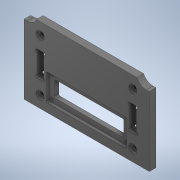
# Autodesk Inventor part: Cockpit_horizontal_frame_05
Saved by Autodesk Inventor 2020.4 (Build 244396000, 396)
## iProperties
Created: 2021-08-14
Part Number: Cockpit_horizontal_frame_05
Material: アセタール樹脂、黒
Document SubType Name: Modeling
Designer: Masato Kubotera
Density: 1.425 g/cm^3
Appearance: 滑らか - 黒
Mass: 37.8231 g
Surface Area: 126.929 cm^2
Volume: 26.5425 cm^3
Description: POM T5
Author: Masato Kubotera
Title: Cockpit_horizontal_frame_05
Autodesk Inventor part; units mm, degrees
ref_plane "YZ Plane" through (0, 0, 0) normal (1, 0, 0) x (0, 1, 0)
ref_plane "XZ Plane" through (0, 0, 0) normal (0, 1, 0) x (-1, 0, 0)
ref_plane "XY Plane" through (0, 0, 0) normal (0, 0, 1) x (1, 0, 0)
sketch "スケッチ1" plane through (0, 0, 0) normal (0, 0, 1) x (1, 0, 0)
  line L0 (-47, 28.25) -> (-37.7144, 28.25)
  line L1 (47, 28.25) -> (47, 23.75)
  line L2 (47, -28.25) -> (-47, -28.25)
  line L3 (-47, -28.25) -> (-47, -11.5167)
  line L4 (-47, 28.25) -> (47, -28.25) construction
  line L5 (47, 28.25) -> (-47, -28.25) construction
  line L6 (0, 28.25) -> (0, -28.25) construction
  line L7 (-47, 11.5167) -> (-47, 23.75)
  line L8 (-47, -11.5167) -> (-47, 11.5167)
  line L9 (47, 11.5167) -> (47, -11.5167)
  line L10 (47, -11.5167) -> (47, -28.25)
  line L11 (-47, 0) -> (47, 0) construction
  arc A0 (-47, 24.0838) -> (-37.7144, 28.25) centre (-44.75, 31.5) ccw
  arc A1 (37.7144, 28.25) -> (47, 24.0838) centre (44.75, 31.5) ccw
  line L12 (-47, 24.0838) -> (-47, 28.25)
  line L13 (-37.7144, 28.25) -> (47, 28.25)
  arc A2 (-37.7144, 28.25) -> (-47, 24.0838) centre (-44.75, 31.5) ccw
  arc A3 (47, 24.0838) -> (37.7144, 28.25) centre (44.75, 31.5) ccw
  line L14 (-44.75, 23.75) -> (-47, 23.75)
  line L15 (44.75, 23.75) -> (47, 23.75)
  line L16 (-47, 23.75) -> (-47, 24.0838)
  line L17 (47, 23.75) -> (47, 11.5167)
  line L18 (-30, -1.75) -> (30, -1.75) construction
  line L19 (30, -1.75) -> (30, -21.75) construction
  line L20 (30, -21.75) -> (-30, -21.75) construction
  line L21 (-30, -21.75) -> (-30, -1.75) construction
  line L22 (-30, -1.75) -> (30, -21.75) construction
  line L23 (30, -1.75) -> (-30, -21.75) construction
  circle A4 centre (-28, -3.75) radius 1.05
  line L24 (30, -11.75) -> (-30, -11.75) construction
  circle A5 centre (-28, -19.75) radius 1.05
  circle A6 centre (28, -3.75) radius 1.05
  circle A7 centre (28, -19.75) radius 1.05
  line L25 (-30.05, -1.7) -> (30.05, -1.7)
  line L26 (30.05, -1.7) -> (30.05, -21.8)
  line L27 (30.05, -21.8) -> (-30.05, -21.8)
  line L28 (-30.05, -21.8) -> (-30.05, -1.7)
  line L29 (-30.05, -1.7) -> (30.05, -21.8) construction
  line L30 (30.05, -1.7) -> (-30.05, -21.8) construction
  line L31 (-26, -5.75) -> (26, -5.75)
  line L32 (26, -5.75) -> (26, -17.75)
  line L33 (26, -17.75) -> (-26, -17.75)
  line L34 (-26, -17.75) -> (-26, -5.75)
  line L35 (-26, -5.75) -> (26, -17.75) construction
  line L36 (26, -5.75) -> (-26, -17.75) construction
  line L37 (-37.25, 9.4167) -> (-32.25, 9.4167) construction
  line L38 (-32.25, 9.4167) -> (-32.25, -9.4167) construction
  line L39 (-32.25, -9.4167) -> (-37.25, -9.4167) construction
  line L40 (-37.25, -9.4167) -> (-37.25, 9.4167) construction
  line L41 (-37.25, 9.4167) -> (-32.25, -9.4167) construction
  line L42 (-32.25, 9.4167) -> (-37.25, -9.4167) construction
  line L43 (-37.26, 9.4267) -> (-32.24, 9.4267)
  line L44 (-32.24, 9.4267) -> (-32.24, 7.3267) construction
  line L45 (-32.24, -9.4267) -> (-37.26, -9.4267)
  line L46 (-37.26, -9.4267) -> (-37.26, -7.3267) construction
  line L47 (-37.26, 9.4267) -> (-32.24, -9.4267) construction
  line L48 (-32.24, 9.4267) -> (-37.26, -9.4267) construction
  arc A8 (-37.26, 9.4267) -> (-37.26, 7.3267) centre (-37.26, 8.3767) ccw
  line L49 (-34.75, 9.4167) -> (-34.75, -9.4167) construction
  line L50 (-37.25, 0) -> (-32.25, 0) construction
  arc A9 (-32.24, 7.3267) -> (-32.24, 9.4267) centre (-32.24, 8.3767) ccw
  arc A10 (-37.26, -7.3267) -> (-37.26, -9.4267) centre (-37.26, -8.3767) ccw
  arc A11 (-32.24, -9.4267) -> (-32.24, -7.3267) centre (-32.24, -8.3767) ccw
  line L51 (-37.26, 7.3267) -> (-37.26, 9.4267) construction
  line L52 (-32.24, 7.3267) -> (-32.24, -7.3267)
  line L53 (-37.26, -7.3267) -> (-37.26, 7.3267)
  line L54 (-32.24, -7.3267) -> (-32.24, -9.4267) construction
  line L55 (37.25, 9.4167) -> (32.25, 9.4167) construction
  line L56 (32.25, 9.4167) -> (32.25, -9.4167) construction
  line L57 (32.25, -9.4167) -> (37.25, -9.4167) construction
  line L58 (37.25, -9.4167) -> (37.25, 9.4167) construction
  line L59 (37.25, 9.4167) -> (32.25, -9.4167) construction
  line L60 (32.25, 9.4167) -> (37.25, -9.4167) construction
  line L61 (37.26, 9.4267) -> (32.24, 9.4267)
  line L62 (32.24, 9.4267) -> (32.24, 7.3267) construction
  line L63 (32.24, -9.4267) -> (37.26, -9.4267)
  line L64 (37.26, -9.4267) -> (37.26, -7.3267) construction
  line L65 (37.26, 9.4267) -> (32.24, -9.4267) construction
  line L66 (32.24, 9.4267) -> (37.26, -9.4267) construction
  arc A12 (37.26, 7.3267) -> (37.26, 9.4267) centre (37.26, 8.3767) ccw
  line L67 (34.75, 9.4167) -> (34.75, -9.4167) construction
  line L68 (37.25, 0) -> (32.25, 0) construction
  arc A13 (32.24, 9.4267) -> (32.24, 7.3267) centre (32.24, 8.3767) ccw
  arc A14 (37.26, -9.4267) -> (37.26, -7.3267) centre (37.26, -8.3767) ccw
  arc A15 (32.24, -7.3267) -> (32.24, -9.4267) centre (32.24, -8.3767) ccw
  line L69 (37.26, 7.3267) -> (37.26, 9.4267) construction
  line L70 (32.24, 7.3267) -> (32.24, -7.3267)
  line L71 (37.26, -7.3267) -> (37.26, 7.3267)
  line L72 (32.24, -7.3267) -> (32.24, -9.4267) construction
  circle A16 centre (-34.75, 19.4167) radius 1.55
  circle A17 centre (-34.75, 19.4167) radius 3
  circle A18 centre (-34.75, -19.4167) radius 1.55
  circle A19 centre (-34.75, -19.4167) radius 3
  circle A20 centre (34.75, 19.4167) radius 1.55
  circle A21 centre (34.75, 19.4167) radius 3
  circle A22 centre (34.75, -19.4167) radius 3
  circle A23 centre (34.75, -19.4167) radius 1.55
  point P0 (0, 0)
  point P1 (0, 0)
  point P2 (0, 0)
  point P3 (0, 0)
  point P4 (0, -11.75)
  point P5 (-34.75, 0)
  point P6 (-34.75, 0)
  point P7 (-34.75, 0)
  point P8 (34.75, 0)
  point P9 (34.75, 0)
  point P10 (34.75, 0)
  point P11 (-34.75, 0)
  dimension "d0" = 94
  dimension "d1" = 56.5
  dimension "d40" = 31.5
  dimension "d41" = 89.5
  dimension "d42" = 15.5
  dimension "d43" = 52
  dimension "d69" = 60
  dimension "d70" = 20
  dimension "d71" = 2
  dimension "d72" = 2
  dimension "d73" = 2.1
  dimension "d74" = 30
  dimension "d75" = 0.05
  dimension "d76" = 0.05
  dimension "d80" = 4
  dimension "d81" = 4
  dimension "d82" = 5
  dimension "d83" = 18.8333
  dimension "d84" = 1.05
  dimension "d87" = 0.01
  dimension "d88" = 0.01
  dimension "d89" = 64.5
  dimension "d90" = 3.1
  dimension "d91" = 6
  dimension "d92" = 10
  constraints: 146 end point, 42 symmetric about line, 40 parallel, 36 midpoint, 26 point on circle, 24 centre point, 17 perpendicular, 9 point on line, 7 horizontal, 4 coincident, 1 tangent, 17 other
  measures "d0" distance of L2.start L2.end
  measures "d1" distance of L2.start L1.start
  measures "d40" vertical distance of L11.start A0.centre
  measures "d41" distance of A1.centre A0.centre
  measures "d42" diameter of A0
  measures "d43" distance of L2.start L1.end
  measures "d69" distance of L19.end L20.end
  measures "d70" distance of L18.end L19.end
  measures "d71" horizontal distance of A4.centre L18.start
  measures "d72" horizontal distance of L18.start A4.centre
  measures "d73" diameter of A4
  measures "d74" distance between parallel lines of L18 L13
  measures "d75" horizontal distance of L25.start L18.start
  measures "d76" horizontal distance of L18.start L25.start
  measures "d80" horizontal distance of L31.start L18.start
  measures "d81" horizontal distance of L31.start L18.start
  measures "d82" distance of L38.end L39.end
  measures "d83" distance of L37.end L38.end
  measures "d84" radius of A8
  measures "d87" distance between parallel lines of L37 L43
  measures "d88" distance between parallel lines of L40 L53
  measures "d89" distance between parallel lines of L38 L56
  measures "d90" diameter of A16
  measures "d91" diameter of A17
  measures "d92" distance of L49.start A17.centre
extrude "押し出し1" add sketch "スケッチ1" along normal blind 5 contours L13 A1 L15 L17 L9 L10 L2 L3 L8 L7 L14 A0
extrude "押し出し2" add sketch "スケッチ1" along normal blind 3 contours L25 L26 L27 L28
fillet "フィレット1" radius 1 8 edges at (-30.05, -1.7, 4) (-30.05, -21.8, 4) (30.05, -21.8, 4) (30.05, -1.7, 4) (-26, -5.75, 1.5) (-26, -17.75, 1.5) (26, -5.75, 1.5) (26, -17.75, 1.5)
extrude "押し出し3" add sketch "スケッチ1" along normal blind 3.5 contours A17 | A19 | A21 | A22
